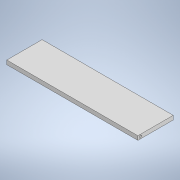
# Autodesk Inventor part: Pala
Saved by Autodesk Inventor 2020.3 (Build 243373000, 373)
## iProperties
Created: 2021-03-20
Part Number: Pala
Material: Generic
Document SubType Name: Modeling
Designer: alexo
Density: 1 g/cm^3
Appearance: Default
Author: alexo
Autodesk Inventor part; units mm, degrees
ref_plane "YZ Plane" through (0, 0, 0) normal (1, 0, 0) x (0, 1, 0)
ref_plane "XZ Plane" through (0, 0, 0) normal (0, 1, 0) x (-1, 0, 0)
ref_plane "XY Plane" through (0, 0, 0) normal (0, 0, 1) x (1, 0, 0)
sketch "Sketch1" plane through (0, 0, 0) normal (0, 1, 0) x (-1, 0, 0)
  line L0 (65, 0) -> (-65, 0)
  line L1 (65, 0) -> (65, 35)
  line L2 (65, 35) -> (-65, 35)
  line L3 (-65, 35) -> (-65, 0)
  point P0 (0, 0)
  point P1 (0, 0)
  dimension "d0" = 130
  dimension "d1" = 35
  constraints: 8 end point, 2 perpendicular, 1 coincident, 1 horizontal, 1 midpoint, 1 vertical
  measures "d0" distance of L0.start L0.end
  measures "d1" distance between parallel lines of L0 L2
extrude "Extrusion1" add sketch "Sketch1" along normal mid plane 4
sketch "Sketch2" plane through (-65, -2, 35) normal (-1, 0, 0) x (0, 0, 1)
  circle A0 centre (-2.5, 2) radius 1.25
  line L0 (0, 0) -> (0, 4) projected
  line L1 (0, 2) -> (-35, 2) construction
  dimension "d4" = 2.5
  dimension "d5" = 2.5
  constraints: 2 end point, 1 centre point, 1 horizontal, 1 midpoint, 1 point on line
  measures "d4" diameter of A0
  measures "d5" distance from line of L0 A0.centre
extrude "Extrusion2" cut sketch "Sketch2" against normal through all
body "Solid1"
